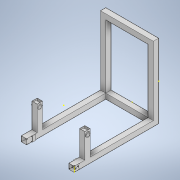
# Autodesk Inventor part: Principal
Saved by Autodesk Inventor 2021 (Build 250183000, 183)
## iProperties
Created: 2022-02-17
Part Number: Principal
Material: Genérico
Document SubType Name: Modeling
Designer: arthu
Density: 1 g/cm^3
Appearance: Valor por defecto
Author: arthu
Autodesk Inventor part; units mm, degrees
ref_plane "YZ Plane" through (0, 0, 0) normal (1, 0, 0) x (0, 1, 0)
ref_plane "XZ Plane" through (0, 0, 0) normal (0, 1, 0) x (-1, 0, 0)
ref_plane "XY Plane" through (0, 0, 0) normal (0, 0, 1) x (1, 0, 0)
sketch "Boceto1" plane through (0, 0, 0) normal (0, 0, 1) x (1, 0, 0)
  line L0 (300, -450) -> (-300, -450)
  line L1 (-300, -450) -> (-300, 450)
  line L2 (-300, 450) -> (300, 450)
  line L3 (300, 450) -> (300, -450)
  line L4 (300, -450) -> (-300, 450) construction
  line L5 (-300, -450) -> (300, 450) construction
  line L6 (376.2, 526.2) -> (-376.2, 526.2)
  line L7 (-376.2, 526.2) -> (-376.2, -526.2)
  line L8 (-376.2, -526.2) -> (376.2, -526.2)
  line L9 (376.2, -526.2) -> (376.2, 526.2)
  line L10 (-300, -450) -> (-300, -526.2)
  line L11 (300, -450) -> (300, -526.2)
  line L12 (300, 450) -> (300, 526.2)
  line L13 (-300, 450) -> (-300, 526.2)
  line L14 (-300, -450) -> (-376.2, -450)
  line L15 (300, -450) -> (376.2, -450)
  point P0 (0, 0)
  dimension "d0" = 600
  dimension "d1" = 900
  dimension "d2" = 76.2
  constraints: 32 end point, 9 point on line, 5 perpendicular, 4 parallel, 2 midpoint, 1 horizontal, 3 other
  measures "d0" distance of L1.end L2.end
  measures "d1" distance of L0.end L1.end
  measures "d2" distance between parallel lines of L2 L6
extrude "Extrusión1" add sketch "Boceto1" along normal blind 76.2 contours L11 L8 L10 L0 | L15 L9 L8 L11 | L3 L12 L6 L9 L15 | L14 L7 L6 L13 L1 | L10 L8 L7 L14 | L2 L13 L6 L12
extrude "Extrusión2" add sketch "Boceto1" along normal blind 1200 contours L15 L9 L8 L11 | L10 L8 L7 L14
sketch "Boceto2" plane through (300, -450, 76.2) normal (0, 1, 0) x (1, 0, 0)
  line L0 (76.2, 0) -> (76.2, -1123.8) projected
  line L1 (76.2, -1123.8) -> (76.2, -973.8)
  line L2 (76.2, -973.8) -> (0, -973.8)
  line L3 (0, 0) -> (0, -1123.8) projected
  line L4 (76.2, -973.8) -> (76.2, -897.6)
  line L5 (76.2, -897.6) -> (0, -897.6)
  line L6 (0, -897.6) -> (0, -973.8)
  line L7 (-600, 0) -> (-600, -1123.8) projected
  line L8 (-600, -897.6) -> (-600, -973.8)
  line L9 (-676.2, 0) -> (-676.2, -1123.8) projected
  line L10 (-676.2, -973.8) -> (-676.2, -897.6)
  line L11 (-600, -897.6) -> (-676.2, -897.6)
  line L12 (-600, -973.8) -> (-676.2, -973.8)
  point P0 (-300, 76.2)
  dimension "d7" = 150
  dimension "d8" = 76.2
  constraints: 18 end point, 11 point on line, 5 perpendicular
  measures "d7" distance of L0.end L1.end
  measures "d8" distance of L1.end L4.end
extrude "Extrusión3" add sketch "Boceto2" along normal blind 350
sketch "Boceto3" plane through (376.2, -526.2, 0) normal (1, 0, 0) x (0, 0, -1)
  line L0 (0, 0) -> (0, 1052.4) projected
  line L1 (0, 1052.4) -> (-76.2, 1052.4) projected
  line L2 (-76.2, 76.2) -> (-76.2, 1052.4) projected
  line L3 (-76.2, 76.2) -> (-973.8, 76.2) projected
  line L4 (-973.8, 76.2) -> (-973.8, 426.2) projected
  line L5 (-1050, 426.2) -> (-973.8, 426.2) projected
  line L6 (-1050, 76.2) -> (-1050, 426.2) projected
  line L7 (-1050, 76.2) -> (-1200, 76.2) projected
  line L8 (-1200, 0) -> (-1200, 76.2) projected
  line L9 (0, 0) -> (-1200, 0) projected
  circle A0 centre (-1011.9, 375.4) radius 25.4
  line L10 (-1011.9, 375.4) -> (-1011.9, 426.2)
  line L11 (-973.8, 426.2) -> (-1050, 426.2) projected
  circle A1 centre (-1011.9, 375.4) radius 25.4
  circle A2 centre (-1011.9, 375.4) radius 33.4
  point P0 (0, 526.2)
  dimension "d11" = 50.8
  dimension "d12" = 50.8
  dimension "d16" = 8
  constraints: 3 centre point, 2 end point, 1 coincident, 1 concentric, 1 midpoint
  measures "d11" diameter of A0
  measures "d12" distance from line of L5 L10.start
  measures "d16" radial gap between concentric circles of A0 A2
extrude "Extrusión4" cut sketch "Boceto3" against normal blind 1200 contours A0
shell "Vaciado1" thickness 2 removed faces 2 at (325.4, -152.8439, 986.5824) at (-350.8, -152.8439, 986.5824)
extrude "Extrusión5" add sketch "Boceto3" against normal blind 76.2 contours A2
sketch "Boceto4" plane through (-376.2, -526.2, 0) normal (-1, 0, 0) x (0, 0, 1)
  circle A0 centre (1011.9, 375.4) radius 33.4 projected
  circle A1 centre (1011.9, 375.4) radius 25.4 projected
  point P0 (0, 526.2)
extrude "Extrusión6" add sketch "Boceto4" against normal blind 76.2
extrude "Extrusión7" add sketch "Boceto3" along normal blind 8.8 contours A2
extrude "Extrusión8" add sketch "Boceto4" along normal blind 8.8
sketch "Boceto5" plane through (376.2, -450, 973.8) normal (0, 0, -1) x (-1, 0, 0)
  point P0 (376.2, 450)
sketch "Boceto6" plane through (0, 0, 1200) normal (0, 0, 1) x (1, 0, 0)
  line L0 (374.2, -452) -> (302, -452) projected
  line L1 (302, -452) -> (302, -524.2) projected
  line L2 (374.2, -524.2) -> (374.2, -452) projected
  line L3 (302, -524.2) -> (374.2, -524.2) projected
  line L4 (300, -526.2) -> (376.2, -526.2) projected
  line L5 (300, -450) -> (300, -526.2) projected
  line L6 (300, -526.2) -> (376.2, -526.2) projected
  line L7 (376.2, -526.2) -> (376.2, -450) projected
  line L8 (376.2, -450) -> (300, -450) projected
  line L9 (-376.2, -450) -> (-376.2, -526.2) projected
  line L10 (-376.2, -526.2) -> (-300, -526.2) projected
  line L11 (-300, -526.2) -> (-300, -450) projected
  line L12 (-300, -450) -> (-376.2, -450) projected
  line L13 (-302, -452) -> (-374.2, -452) projected
  line L14 (-302, -524.2) -> (-302, -452) projected
  line L15 (-374.2, -452) -> (-374.2, -524.2) projected
  line L16 (-374.2, -524.2) -> (-302, -524.2) projected
  point P0 (0, 0)
extrude "Extrusión9" cut sketch "Boceto6" against normal blind 2 contours L2 L3 L1 L0 | L14 L16 L15 L13
sketch "Boceto7" plane through (300, -100, 76.2) normal (0, 1, 0) x (1, 0, 0)
  line L0 (-600, -973.8) -> (-600, -897.6) projected
  line L1 (-600, -897.6) -> (-676.2, -897.6) projected
  line L2 (-676.2, -897.6) -> (-676.2, -973.8) projected
  line L3 (-676.2, -973.8) -> (-600, -973.8) projected
  line L4 (-674.2, -899.6) -> (-674.2, -971.8) projected
  line L5 (-674.2, -971.8) -> (-602, -971.8) projected
  line L6 (-602, -899.6) -> (-674.2, -899.6) projected
  line L7 (-602, -971.8) -> (-602, -899.6) projected
  line L8 (0, -897.6) -> (0, -973.8) projected
  line L9 (0, -973.8) -> (76.2, -973.8) projected
  line L10 (76.2, -973.8) -> (76.2, -897.6) projected
  line L11 (76.2, -897.6) -> (0, -897.6) projected
  line L12 (2, -899.6) -> (2, -971.8) projected
  line L13 (2, -971.8) -> (74.2, -971.8) projected
  line L14 (74.2, -899.6) -> (2, -899.6) projected
  line L15 (74.2, -971.8) -> (74.2, -899.6) projected
  point P0 (-300, 76.2)
extrude "Extrusión10" cut sketch "Boceto7" against normal blind 2 contours L6 L7 L5 L4 | L14 L15 L13 L12
sketch "Boceto8" plane through (-376.2, -450, 1200) normal (0, 1, 0) x (1, 0, 0)
  point P0 (376.2, 1200)
sketch "Boceto9" plane through (376.2, -526.2, 0) normal (1, 0, 0) x (0, 0, -1)
  line L0 (-1200, 74.2) -> (-1200, 2) projected
  line L1 (-1200, 38.1) -> (-1174.6, 38.1)
  point P0 (0, 526.2)
  dimension "d29" = 25.4
  constraints: 2 end point, 1 horizontal, 1 midpoint
  measures "d29" distance of L1.start L1.end
ref_plane "Plano de trabajo1" through (0, -526.2, 0) normal (1, 0, 0) x (0, 0, -1)
sketch "Boceto12" plane through (376.2, -526.2, 0) normal (1, 0, 0) x (0, 0, -1)
  line L0 (0, 0) -> (-1200, 0) projected
  line L1 (-1050, 76.2) -> (-1200, 76.2) projected
  line L2 (-1200, 0) -> (-1123.8, 0)
  line L3 (-1123.8, 0) -> (-1123.8, 76.2)
  line L4 (-1123.8, 76.2) -> (-1200, 76.2)
  line L5 (-1200, 76.2) -> (-1200, 0)
  circle A0 centre (-1192.6591, 7.3409) radius 4
  circle A1 centre (-1131.1409, 7.3409) radius 4
  circle A2 centre (-1131.1409, 68.8591) radius 4
  circle A3 centre (-1192.6591, 68.8591) radius 4
  point P0 (0, 526.2)
  dimension "d30" = 76.2
  dimension "d32" = 8
  dimension "d33" = 8
  dimension "d34" = 8
  dimension "d35" = 8
  constraints: 8 end point, 4 centre point, 2 parallel, 1 horizontal, 1 perpendicular, 1 point on line
  measures "d30" distance of L4.end L3.end
  measures "d32" diameter of A0
  measures "d33" diameter of A1
  measures "d34" diameter of A2
  measures "d35" diameter of A3
extrude "Extrusión11" cut sketch "Boceto12" against normal blind 770 contours A0 | A1 | A2 | A3
sketch "Boceto13" plane through (-300, -526.2, 76.2) normal (1, 0, 0) x (0, 0, -1)
  line L0 (-1123.8, 76.2) -> (-1123.8, 0) projected
  line L1 (-973.8, 76.2) -> (-1123.8, 76.2) projected
  line L2 (-1123.8, 0) -> (-1047.6, 0)
  line L3 (-1047.6, 0) -> (-1047.6, 76.2)
  line L4 (-1047.6, 76.2) -> (-1123.8, 76.2)
  line L5 (-1123.8, 76.2) -> (-1123.8, 0)
  line L6 (-973.8, 76.2) -> (-1123.8, 76.2) projected
  line L7 (-1047.6, 0) -> (-1007.6, 0)
  line L8 (-1007.6, 0) -> (-1007.6, 76.2)
  line L9 (-1007.6, 76.2) -> (-1047.6, 76.2)
  line L10 (-1047.6, 76.2) -> (-1047.6, 0)
  point P0 (76.2, 526.2)
  point P1 (-1007.6, 76.2)
  dimension "d38" = 76.2
  dimension "d39" = 40
  constraints: 16 end point, 4 parallel, 2 horizontal, 2 perpendicular, 2 point on line
  measures "d38" distance of L4.end L3.end
  measures "d39" distance of L9.end L8.end
extrude "Extrusión12" add sketch "Boceto13" along normal blind 8 contours L1 L8 L7 L3
sketch "Boceto14" plane through (300, -526.2, 76.2) normal (-1, 0, 0) x (0, 0, 1)
  line L0 (1007.6, 76.2) -> (1007.6, 0) projected
  line L1 (1047.6, 0) -> (1047.6, 76.2) projected
  circle A0 centre (1054.9409, 68.8591) radius 4 projected
  circle A1 centre (1054.9409, 7.3409) radius 4 projected
  circle A2 centre (1116.4591, 68.8591) radius 4 projected
  circle A3 centre (1116.4591, 7.3409) radius 4 projected
  circle A4 centre (935.7, 375.4) radius 25.4 projected
  line L2 (0, 0) -> (0, 76.2) projected
  line L3 (0, 0) -> (1123.8, 0) projected
  line L4 (1123.8, 76.2) -> (1123.8, 0) projected
  line L5 (973.8, 76.2) -> (1123.8, 76.2) projected
  line L6 (973.8, 76.2) -> (973.8, 426.2) projected
  line L7 (897.6, 426.2) -> (973.8, 426.2) projected
  line L8 (897.6, 76.2) -> (897.6, 426.2) projected
  line L9 (0, 76.2) -> (897.6, 76.2) projected
  point P0 (-76.2, 526.2)
extrude "Extrusión13" add sketch "Boceto14" along normal blind 8 contours L5 L1 L3 L0
